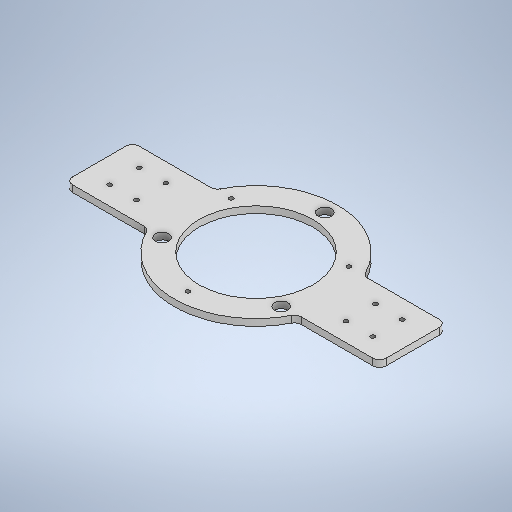
# Autodesk Inventor part: Metal Head Thing
Saved by Autodesk Inventor 2025 (Build 290162000, 162)
## iProperties
Created: 2025-02-06
Part Number: Metal Head Thing
Material: Generic
Document SubType Name: Modeling
Designer: mayhe
Density: 1 g/cm^3
Appearance: Default
Author: mayhe
Autodesk Inventor part; units mm, degrees
ref_plane "YZ Plane" through (0, 0, 0) normal (1, 0, 0) x (0, 1, 0)
ref_plane "XZ Plane" through (0, 0, 0) normal (0, 1, 0) x (-1, 0, 0)
ref_plane "XY Plane" through (0, 0, 0) normal (0, 0, 1) x (1, 0, 0)
sketch "Sketch1" plane through (0, 0, 0) normal (0, 1, 0) x (-1, 0, 0)
  circle A0 centre (0, 0) radius 42.5
  arc A1 (55.6417, 25) -> (-55.6417, 25) centre (0, 0) ccw
  line L0 (0, 0) -> (0, -61)
  line L1 (0, 0) -> (0, 0)
  line L2 (0, 0) -> (0, -90.4875)
  line L3 (-117.5, 25) -> (-117.5, -25)
  line L4 (117.5, -25) -> (117.5, 25)
  line L5 (117.5, 25) -> (-117.5, -25) construction
  line L6 (-117.5, 25) -> (117.5, -25) construction
  line L7 (117.5, 25) -> (55.6417, 25)
  line L8 (-55.6417, 25) -> (-117.5, 25)
  line L9 (55.6417, -25) -> (117.5, -25)
  line L10 (-117.5, -25) -> (-55.6417, -25)
  arc A2 (-55.6417, -25) -> (55.6417, -25) centre (0, 0) ccw
  dimension "d0" = 85
  dimension "d29" = 61
  dimension "d46" = 235
  dimension "d47" = 50
  constraints: 22 end point, 5 parallel, 4 coincident, 4 point on circle, 3 centre point, 3 horizontal, 2 midpoint, 2 perpendicular, 2 vertical, 1 point on line, 1 vertical alignment
  measures "d0" diameter of A0
  measures "d29" radius of A1
  measures "d46" distance of L4.start L3.end
  measures "d47" distance of L3.end L3.start
extrude "Extrusion1" add sketch "Sketch1" along normal blind 5
sketch "Sketch2" plane through (0, 0, 0) normal (0, -1, 0) x (1, 0, 0)
  line L0 (-117.5, -25) -> (-117.5, 25) projected
  line L1 (-117.5, 0) -> (117.5, 0)
  line L2 (117.5, 25) -> (117.5, -25) projected
  arc A0 (55.6417, 25) -> (-55.6417, 25) centre (0, 0) ccw projected
  line L3 (0, 61) -> (0, -61)
  arc A1 (-55.6417, -25) -> (55.6417, -25) centre (0, 0) ccw projected
  circle A2 centre (-98.5, 11) radius 2
  line L4 (-117.5, 25) -> (-55.6417, 25) projected
  circle A3 centre (-78.5, 11) radius 2
  circle A4 centre (-98.5, -11) radius 2
  circle A5 centre (-78.5, -11) radius 2
  circle A6 centre (98.5, 11) radius 2
  circle A7 centre (78.5, 11) radius 2
  circle A8 centre (98.5, -11) radius 2
  circle A9 centre (78.5, -11) radius 2
  dimension "d51" = 4
  dimension "d52" = 19
  dimension "d53" = 14
  dimension "d54" = 4
  dimension "d55" = 20
  constraints: 8 centre point, 6 symmetric about line, 4 end point, 2 midpoint, 2 point on circle, 1 perpendicular, 6 other
  measures "d51" diameter of A2
  measures "d52" distance from line of L0 A2.centre
  measures "d53" distance from line of L4 A2.centre
  measures "d54" diameter of A3
  measures "d55" distance of A3.centre A2.centre
hole "Hole1" at (-98.5, 0, 11) at (-78.5, 0, 11) at (-78.5, 0, -11) at (-98.5, 0, -11) at (78.5, 0, 11) at (98.5, 0, 11) at (98.5, 0, -11) at (78.5, 0, -11) direction (0, 1, 0) diameter 3.242 depth 11.8 tip angle 118 thread size "M4x0.7" class "6H" standard "ANSI Metric M Profile"
fillet "Fillet2" radius 5 8 edges at (-117.5, 2.5, -25) (-55.6417, 2.5, -25) (117.5, 2.5, -25) (55.6417, 2.5, -25) (117.5, 2.5, 25) (55.6417, 2.5, 25) (-55.6417, 2.5, 25) (-117.5, 2.5, 25)
sketch "Sketch4" plane through (0, 5, 0) normal (0, 1, 0) x (1, 0, 0)
  circle A0 centre (0, 0) radius 51.5
  point P0 (0, 51.5)
  point P1 (-44.6003, -25.75)
  point P2 (44.6003, -25.75)
  dimension "d57" = 103
  dimension "d60" = 360
  constraints: 1 coincident, 1 vertical alignment, 6 other
hole "Pins" at (0, 5, -51.5) at (-44.6003, 5, 25.75) at (44.6003, 5, 25.75) direction (0, -1, 0) diameter 10 end through all
sketch "Sketch5" plane through (0, 5, 0) normal (0, 1, 0) x (1, 0, 0)
  circle A0 centre (0, 0) radius 51
  point P0 (0, -51)
  point P1 (0, -51)
  dimension "d69" = 102
  constraints: 2 coincident, 1 vertical alignment, 2 other
hole "Mounting Holes" at (0, 5, 51) direction (0, -1, 0) diameter 3.242 end through all thread size "M4x0.7" class "6H" standard "ANSI Metric M Profile"
pattern_circular "Circular Pattern1" count 3 over 360 about axis through (0, -10, 0) along (0, 1, 0) of "Mounting Holes"
body "Solid1"
